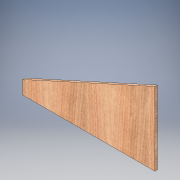
# Autodesk Inventor part: verticalff1
Saved by Autodesk Inventor 2019 (Build 230136000, 136)
## iProperties
Created: 2019-01-07
Part Number: verticalff1
Material: Wood (Birch)
Document SubType Name: Modeling
Designer: gaincarlo
Density: 0.55 g/cm^3
Appearance: Birch - Natural Polished
Author: gaincarlo
Autodesk Inventor part; units mm, degrees
ref_plane "YZ Plane" through (0, 0, 0) normal (1, 0, 0) x (0, 1, 0)
ref_plane "XZ Plane" through (0, 0, 0) normal (0, 1, 0) x (-1, 0, 0)
ref_plane "Work Plane1" through (0, 0, 0) normal (0, 0, 1) x (1, 0, 0)
sketch "Sketch1" plane through (0, 0, 0) normal (0, 0, 1) x (1, 0, 0)
  line L0 (-560, 55) -> (-11.1724, 304.4671) construction
  line L1 (-10.3448, 302.6464) -> (-559.1724, 53.1793)
  line L2 (-559.1724, 53.1793) -> (-560, 55)
  line L3 (-10, 600) -> (0, 600) construction
  line L4 (0, 600) -> (0, 0) construction
  line L5 (0, 0) -> (-10, 0) construction
  line L6 (-10, 0) -> (-10, 600) construction
  line L7 (-10, 17.7053) -> (-559.1724, 17.7053)
  line L8 (-559.1724, 53.1793) -> (-559.1724, 17.7053)
  line L9 (-559.1724, 17.7053) -> (-10, 17.7053)
  line L10 (-10, 17.7053) -> (-10, 0)
  line L11 (-10, 0) -> (-559.1724, 0)
  line L12 (-559.1724, 0) -> (-559.1724, 17.7053)
  line L13 (-10, 302.6464) -> (-10.3448, 302.6464)
  line L14 (-10, 17.7053) -> (-10, 302.6464)
  point P0 (-10, 202.6464)
  constraints: 30 end point, 5 horizontal, 3 perpendicular, 2 parallel, 2 vertical, 1 point on line, 12 other
extrude "Extrusion5" add sketch "Sketch1" along normal mid plane 10
sketch "Sketch2" plane through (0, 0, 5) normal (0, 0, 1) x (1, 0, 0)
  line L0 (-559.1724, 53.1793) -> (-559.1724, 0) projected
  line L1 (-559.1724, 0) -> (-555.1724, 0)
  line L2 (-555.1724, 0) -> (-555.1724, 80)
  line L3 (-555.1724, 80) -> (-559.1724, 80)
  line L4 (-559.1724, 80) -> (-559.1724, 0)
  point P0 (0, 0)
  dimension "d10" = 4
  dimension "d11" = 80
  constraints: 8 end point, 2 parallel, 1 horizontal, 1 perpendicular
  measures "d10" distance of L3.end L2.end
  measures "d11" distance of L2.end L1.end
extrude "Extrusion6" cut sketch "Sketch2" against normal through all
body "Solid2"
